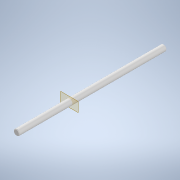
# Autodesk Inventor part: ryrka2
Saved by Autodesk Inventor 2021 (Build 250183000, 183)
## iProperties
Created: 2021-06-18
Part Number: ryrka2
Material: Ogólny
Document SubType Name: Modeling
Designer: Wojciech Wołczek
Density: 1 g/cm^3
Appearance: Domyślna
Author: Wojciech Wołczek
Autodesk Inventor part; units mm, degrees
ref_plane "YZ Plane" through (0, 0, 0) normal (1, 0, 0) x (0, 1, 0)
ref_plane "XZ Plane" through (0, 0, 0) normal (0, 1, 0) x (-1, 0, 0)
ref_plane "XY Plane" through (0, 0, 0) normal (0, 0, 1) x (1, 0, 0)
ref_plane "Płaszczyzna konstrukcyjna1" through (-0.1106, 0.0064, 0) normal (0, 0, 1) x (1, 0, 0)
sketch "Szkic1" plane through (-0.1106, 0.0064, 0) normal (0, 0, 1) x (1, 0, 0)
  circle A0 centre (27.6196, -15.0064) radius 10 projected
  circle A1 centre (27.6196, -15.0064) radius 10
  point P0 (0.1106, -0.0064)
  dimension "d0" = 20
  constraints: 1 centre point, 1 coincident
  measures "d0" diameter of A1
extrude "Wyciągnięcie proste1" add sketch "Szkic1" along normal blind 180 and the other way blind 320
chamfer "Faza1" distance 2 angle 45 2 edges at (17.509, -15, 180) (17.509, -15, -320)
